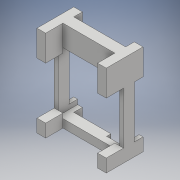
# Autodesk Inventor part: 140mmLaptopStand
Saved by Autodesk Inventor 2017 (Build 210142000, 142)
## iProperties
Created: 2016-09-13
Part Number: 140mmLaptopStand
Material: Generic
Document SubType Name: Modeling
Designer: Schmidty15
Density: 1 g/cm^3
Appearance: Default
Author: Schmidty15
Autodesk Inventor part; units mm, degrees
ref_plane "YZ Plane" through (0, 0, 0) normal (1, 0, 0) x (0, 1, 0)
ref_plane "XZ Plane" through (0, 0, 0) normal (0, 1, 0) x (-1, 0, 0)
ref_plane "XY Plane" through (0, 0, 0) normal (0, 0, 1) x (1, 0, 0)
sketch "Sketch1" plane through (0, 0, 0) normal (0, 1, 0) x (-1, 0, 0)
  line L0 (0, 0) -> (-160, 0)
  line L1 (-160, 0) -> (-160, 190)
  line L2 (-160, 190) -> (0, 190)
  line L3 (0, 190) -> (0, 0)
  dimension "d0" = 160
  dimension "d1" = 190
  constraints: 8 end point, 2 parallel, 1 horizontal, 1 perpendicular
  measures "d0" distance of L1.end L2.end
  measures "d1" distance of L0.end L1.end
extrude "Extrusion1" add sketch "Sketch1" along normal blind 55
sketch "Sketch2" plane through (0, 55, 0) normal (0, 1, 0) x (1, 0, 0)
  line L0 (0, 0) -> (10, 0)
  line L1 (10, 0) -> (10, -10)
  line L2 (10, -10) -> (0, -10)
  line L3 (0, -10) -> (0, 0)
  line L4 (10, -10) -> (150, -10)
  line L5 (150, -10) -> (150, -150)
  line L6 (150, -150) -> (10, -150)
  line L7 (10, -150) -> (10, -10)
  dimension "d4" = 10
  dimension "d5" = 10
  dimension "d6" = 140
  dimension "d7" = 140
  constraints: 16 end point, 4 parallel, 2 horizontal, 2 perpendicular
  measures "d4" distance of L1.end L2.end
  measures "d5" distance of L0.end L1.end
  measures "d6" distance of L5.end L6.end
  measures "d7" distance of L4.end L5.end
extrude "Extrusion2" cut sketch "Sketch2" against normal blind 35 contours L4 L5 L6 L7
sketch "Sketch3" plane through (0, 20, 0) normal (0, 1, 0) x (1, 0, 0)
  line L0 (10, -150) -> (10, -10) projected
  line L1 (10, -10) -> (20, -10)
  line L2 (20, -10) -> (20, -20)
  line L3 (20, -20) -> (10, -20)
  line L4 (10, -20) -> (10, -10)
  line L5 (20, -20) -> (140, -20)
  line L6 (140, -20) -> (140, -140)
  line L7 (140, -140) -> (20, -140)
  line L8 (20, -140) -> (20, -20)
  point P0 (0, 0)
  dimension "d10" = 10
  dimension "d11" = 10
  dimension "d12" = 120
  dimension "d13" = 120
  constraints: 16 end point, 4 parallel, 2 horizontal, 2 perpendicular
  measures "d10" distance of L2.end L3.end
  measures "d11" distance of L1.end L2.end
  measures "d12" distance of L6.end L7.end
  measures "d13" distance of L5.end L6.end
extrude "Extrusion3" cut sketch "Sketch3" against normal blind 20 contours L5 L6 L7 L8
sketch "Sketch4" plane through (0, 20, 0) normal (0, 1, 0) x (1, 0, 0)
  line L0 (20, -20) -> (20, -140) projected
  line L1 (20, -20) -> (10, -20)
  line L2 (10, -20) -> (10, -140)
  line L3 (10, -140) -> (20, -140)
  line L4 (20, -140) -> (20, -20)
  line L5 (140, -20) -> (20, -20) projected
  line L6 (140, -20) -> (150, -20)
  line L7 (150, -20) -> (150, -140)
  line L8 (150, -140) -> (140, -140)
  line L9 (140, -140) -> (140, -20)
  line L10 (20, -20) -> (140, -20)
  line L11 (140, -20) -> (140, -10)
  line L12 (140, -10) -> (20, -10)
  line L13 (20, -10) -> (20, -20)
  line L14 (20, -140) -> (140, -140)
  line L15 (140, -140) -> (140, -150)
  line L16 (140, -150) -> (20, -150)
  line L17 (20, -150) -> (20, -140)
  point P0 (0, 0)
  dimension "d16" = 10
  dimension "d17" = 10
  dimension "d18" = 120
  dimension "d19" = 120
  dimension "d20" = 10
  dimension "d21" = 120
  dimension "d22" = 10
  constraints: 32 end point, 8 parallel, 4 horizontal, 4 perpendicular
  measures "d16" distance of L3.end L2.end
  measures "d17" distance of L7.end L8.end
  measures "d18" distance of L6.end L7.end
  measures "d19" distance of L12.end L11.end
  measures "d20" distance of L11.end L10.end
  measures "d21" distance of L15.end L16.end
  measures "d22" distance of L14.end L15.end
extrude "Extrusion4" cut sketch "Sketch4" against normal blind 20 contours L0 L3 L2 L1 | L13 L12 L11 L5 | L14 L15 L16 L17 | L6 L7 L8 L9
sketch "Sketch5" plane through (10, 55, 150) normal (1, 0, 0) x (0, 0, -1)
  line L0 (0, -35) -> (10, -35) projected
  line L1 (10, -35) -> (130, -35)
  line L2 (130, -35) -> (130, -55)
  line L3 (130, -55) -> (10, -55)
  line L4 (10, -55) -> (10, -35)
  point P0 (150, -55)
  constraints: 8 end point, 2 parallel, 1 horizontal, 1 perpendicular
extrude "Extrusion5" cut sketch "Sketch5" against normal blind 10
sketch "Sketch6" plane through (150, 55, 10) normal (-1, 0, 0) x (0, 0, 1)
  line L0 (130, -35) -> (130, -55) projected
  line L1 (10, -35) -> (130, -35)
  line L2 (130, -35) -> (130, -55)
  line L3 (130, -55) -> (10, -55)
  line L4 (10, -55) -> (10, -35)
  point P0 (-10, -55)
  dimension "d27" = 120
  dimension "d28" = 20
  constraints: 8 end point, 2 parallel, 1 horizontal, 1 perpendicular
  measures "d27" distance of L0.end L3.end
  measures "d28" distance of L1.end L0.end
extrude "Extrusion6" cut sketch "Sketch6" against normal blind 10
sketch "Sketch7" plane through (0, 0, 0) normal (0, -1, 0) x (1, 0, 0)
  line L0 (160, 190) -> (0, 190) projected
  line L1 (160, 190) -> (150, 190)
  line L2 (150, 190) -> (150, 180)
  line L3 (150, 180) -> (160, 180)
  line L4 (160, 180) -> (160, 190)
  line L5 (0, 140) -> (20, 140) projected
  line L6 (150, 150) -> (10, 150) projected
  line L7 (0, 140) -> (20, 140)
  line L8 (20, 140) -> (20, 150)
  line L9 (20, 150) -> (0, 150)
  line L10 (0, 150) -> (0, 140)
  line L11 (10, 150) -> (10, 10) projected
  line L12 (10, 150) -> (20, 150)
  line L13 (20, 150) -> (20, 160)
  line L14 (20, 160) -> (10, 160)
  line L15 (10, 160) -> (10, 150)
  line L16 (10, 160) -> (150, 160)
  line L17 (150, 160) -> (150, 180)
  line L18 (150, 180) -> (10, 180)
  line L19 (10, 180) -> (10, 160)
  point P0 (0, 0)
  dimension "d31" = 10
  dimension "d32" = 10
  dimension "d33" = 20
  dimension "d34" = 10
  dimension "d35" = 10
  constraints: 32 end point, 8 parallel, 4 horizontal, 4 perpendicular, 1 point on line
  measures "d31" distance of L3.end L2.end
  measures "d32" distance of L2.end L1.end
  measures "d33" distance of L9.end L8.end
  measures "d34" distance of L14.end L13.end
  measures "d35" distance of L13.end L12.end
extrude "Extrusion7" cut sketch "Sketch7" against normal blind 45 contours L17 L16 L14 L19 L18
sketch "Sketch8" plane through (10, 55, 10) normal (0, 0, 1) x (1, 0, 0)
  line L0 (10, -35) -> (10, -55) projected
  line L1 (130, -55) -> (10, -55)
  line L2 (10, -55) -> (10, -35)
  line L3 (10, -35) -> (130, -35)
  line L4 (130, -35) -> (130, -55)
  point P0 (-10, -55)
  dimension "d38" = 120
  dimension "d39" = 20
  constraints: 8 end point, 2 parallel, 1 horizontal, 1 perpendicular
  measures "d38" distance of L0.start L3.end
  measures "d39" distance of L1.end L0.start
extrude "Extrusion8" cut sketch "Sketch8" against normal blind 10
sketch "Sketch9" plane through (150, 55, 10) normal (-1, 0, 0) x (0, 0, 1)
  line L0 (140, 0) -> (140, -35) projected
  line L1 (0, 0) -> (0, -35) projected
  line L2 (140, -35) -> (0, -35)
  line L3 (0, -35) -> (0, 0)
  line L4 (0, 0) -> (140, 0)
  line L5 (140, 0) -> (140, -35)
  point P0 (-10, -55)
  constraints: 8 end point, 2 parallel, 1 horizontal, 1 perpendicular
extrude "Extrusion9" cut sketch "Sketch9" against normal blind 1
sketch "Sketch10" plane through (10, 55, 150) normal (1, 0, 0) x (0, 0, -1)
  line L0 (0, 0) -> (0, -35) projected
  line L1 (0, 0) -> (140, 0)
  line L2 (140, 0) -> (140, -35)
  line L3 (140, -35) -> (0, -35)
  line L4 (0, -35) -> (0, 0)
  point P0 (150, -55)
  constraints: 8 end point, 2 parallel, 1 horizontal, 1 perpendicular
extrude "Extrusion10" cut sketch "Sketch10" against normal blind 1
sketch "Sketch11" plane through (20, 20, 10) normal (0, 0, 1) x (1, 0, 0)
  line L0 (120, 0) -> (131, 0) projected
  line L1 (131, 0) -> (-11, 0)
  line L2 (-11, 0) -> (-11, 35)
  line L3 (-11, 35) -> (131, 35)
  line L4 (131, 35) -> (131, 0)
  point P0 (-20, -20)
  constraints: 8 end point, 2 parallel, 1 horizontal, 1 perpendicular
extrude "Extrusion11" cut sketch "Sketch11" against normal blind 1
sketch "Sketch12" plane through (140, 0, 150) normal (0, 0, -1) x (-1, 0, 0)
  line L0 (-11, 55) -> (-11, 20) projected
  line L1 (-11, 55) -> (131, 55)
  line L2 (131, 55) -> (131, 20)
  line L3 (131, 20) -> (-11, 20)
  line L4 (-11, 20) -> (-11, 55)
  line L5 (0, 0) -> (-20, 0) projected
  line L6 (0, 0) -> (120, 0)
  line L7 (120, 0) -> (120, 20)
  line L8 (120, 20) -> (0, 20)
  line L9 (0, 20) -> (0, 0)
  point P0 (140, 0)
  constraints: 16 end point, 4 parallel, 2 horizontal, 2 perpendicular
extrude "Extrusion12" cut sketch "Sketch12" against normal blind 1
sketch "Sketch14" plane through (160, 55, 0) normal (0, 0, -1) x (-1, 0, 0)
  line L0 (0, -55) -> (0, 0) projected
  line L1 (20, -35) -> (20, -55) projected
  line L2 (0, -55) -> (20, -55)
  line L3 (20, -55) -> (20, -35)
  line L4 (20, -35) -> (0, -35)
  line L5 (0, -35) -> (0, -55)
  line L6 (160, -55) -> (160, -35) projected
  line L7 (140, -35) -> (140, -55) projected
  line L8 (160, -55) -> (140, -55)
  line L9 (140, -55) -> (140, -35)
  line L10 (140, -35) -> (160, -35)
  line L11 (160, -35) -> (160, -55)
  line L12 (151, -35) -> (160, -35) projected
  line L13 (160, 0) -> (0, 0) projected
  line L14 (160, -35) -> (0, -35)
  line L15 (0, -35) -> (0, 0)
  line L16 (0, 0) -> (160, 0)
  line L17 (160, 0) -> (160, -35)
  constraints: 24 end point, 6 parallel, 3 horizontal, 3 perpendicular
extrude "Extrusion13" add sketch "Sketch14" along normal blind 10
sketch "Sketch15" plane through (0, 0, 190) normal (0, 0, 1) x (1, 0, 0)
  line L0 (0, 0) -> (0, 55) projected
  line L1 (160, 0) -> (140, 0) projected
  line L2 (0, 55) -> (160, 55)
  line L3 (160, 55) -> (160, 0)
  line L4 (160, 0) -> (0, 0)
  line L5 (0, 0) -> (0, 55)
  constraints: 8 end point, 2 parallel, 1 horizontal, 1 perpendicular
extrude "Extrusion14" add sketch "Sketch15" along normal blind 10
sketch "Sketch16" plane through (0, 45, 0) normal (0, -1, 0) x (1, 0, 0)
  line L0 (10, 160) -> (10, 180) projected
  line L1 (10, 180) -> (150, 180) projected
  line L2 (10, 160) -> (150, 160)
  line L3 (150, 160) -> (150, 180)
  line L4 (150, 180) -> (10, 180)
  line L5 (10, 180) -> (10, 160)
  point P0 (0, 0)
  constraints: 8 end point, 2 parallel, 1 horizontal, 1 perpendicular
extrude "Extrusion15" add sketch "Sketch16" along normal blind 45
sketch "Sketch17" plane through (20, 20, 9) normal (0, 0, 1) x (1, 0, 0)
  line L0 (-11, 0) -> (-11, 35) projected
  line L1 (-11, 35) -> (131, 35)
  line L2 (131, 35) -> (131, 25)
  line L3 (131, 25) -> (-11, 25)
  line L4 (-11, 25) -> (-11, 35)
  point P0 (-20, -20)
  dimension "d56" = 142
  dimension "d57" = 10
  constraints: 8 end point, 2 parallel, 1 horizontal, 1 perpendicular
  measures "d56" distance of L2.end L3.end
  measures "d57" distance of L1.end L2.end
extrude "Extrusion16" cut sketch "Sketch17" against normal blind 19
sketch "Sketch19" plane through (9, 55, 150) normal (1, 0, 0) x (0, 0, -1)
  line L0 (160, 0) -> (160, -10) projected
  line L1 (141, -10) -> (160, -10) projected
  line L2 (160, 0) -> (141, 0)
  line L3 (141, 0) -> (141, -10)
  line L4 (141, -10) -> (160, -10)
  line L5 (160, -10) -> (160, 0)
  point P0 (150, -55)
  constraints: 8 end point, 2 parallel, 1 horizontal, 1 perpendicular
extrude "Extrusion17" add sketch "Sketch19" along normal blind 11
sketch "Sketch21" plane through (151, 55, 10) normal (-1, 0, 0) x (0, 0, 1)
  line L0 (-20, -10) -> (-20, 0) projected
  line L1 (-1, -10) -> (-1, -35) projected
  line L2 (-20, 0) -> (-1, 0)
  line L3 (-1, 0) -> (-1, -10)
  line L4 (-1, -10) -> (-20, -10)
  line L5 (-20, -10) -> (-20, 0)
  point P0 (-10, -55)
  constraints: 8 end point, 2 parallel, 1 horizontal, 1 perpendicular
extrude "Extrusion18" add sketch "Sketch21" along normal blind 11
sketch "Sketch22" plane through (151, 55, 10) normal (-1, 0, 0) x (0, 0, 1)
  line L0 (-1, 0) -> (141, 0) projected
  line L1 (-1, 0) -> (141, 0)
  line L2 (141, 0) -> (141, -10)
  line L3 (141, -10) -> (-1, -10)
  line L4 (-1, -10) -> (-1, 0)
  point P0 (-10, -55)
  dimension "d64" = 142
  dimension "d65" = 10
  constraints: 8 end point, 2 parallel, 1 horizontal, 1 perpendicular
  measures "d64" distance of L2.end L3.end
  measures "d65" distance of L1.end L2.end
extrude "Extrusion19" cut sketch "Sketch22" against normal blind 9
sketch "Sketch23" plane through (20, 20, 9) normal (0, 0, 1) x (1, 0, 0)
  line L0 (120, 35) -> (140, 35) projected
  line L1 (131, 25) -> (140, 25) projected
  line L2 (140, 35) -> (131, 35)
  line L3 (131, 35) -> (131, 25)
  line L4 (131, 25) -> (140, 25)
  line L5 (140, 25) -> (140, 35)
  point P0 (-20, -20)
  constraints: 8 end point, 2 parallel, 1 horizontal, 1 perpendicular
extrude "Extrusion20" add sketch "Sketch23" along normal blind 11
sketch "Sketch24" plane through (9, 55, 150) normal (1, 0, 0) x (0, 0, -1)
  line L0 (-1, 0) -> (141, 0) projected
  line L1 (141, 0) -> (-1, 0)
  line L2 (-1, 0) -> (-1, -10)
  line L3 (-1, -10) -> (141, -10)
  line L4 (141, -10) -> (141, 0)
  point P0 (150, -55)
  dimension "d70" = 142
  dimension "d71" = 10
  constraints: 8 end point, 2 parallel, 1 horizontal, 1 perpendicular
  measures "d70" distance of L3.end L2.end
  measures "d71" distance of L2.end L1.end
extrude "Extrusion21" cut sketch "Sketch24" against normal blind 9
sketch "Sketch25" plane through (20, 20, 9) normal (0, 0, 1) x (1, 0, 0)
  line L0 (-20, 25) -> (-20, 35) projected
  line L1 (-11, 0) -> (-11, 25) projected
  line L2 (-20, 35) -> (-11, 35)
  line L3 (-11, 35) -> (-11, 25)
  line L4 (-11, 25) -> (-20, 25)
  line L5 (-20, 25) -> (-20, 35)
  point P0 (-20, -20)
  constraints: 8 end point, 2 parallel, 1 horizontal, 1 perpendicular
extrude "Extrusion22" add sketch "Sketch25" along normal blind 11
sketch "Sketch26" plane through (140, 0, 151) normal (0, 0, -1) x (-1, 0, 0)
  line L0 (-20, 45) -> (-20, 55) projected
  line L1 (-11, 45) -> (-20, 45) projected
  line L2 (-20, 55) -> (-11, 55)
  line L3 (-11, 55) -> (-11, 45)
  line L4 (-11, 45) -> (-20, 45)
  line L5 (-20, 45) -> (-20, 55)
  line L6 (-20, 55) -> (140, 55) projected
  line L7 (131, 45) -> (140, 45) projected
  line L8 (140, 55) -> (131, 55)
  line L9 (131, 55) -> (131, 45)
  line L10 (131, 45) -> (140, 45)
  line L11 (140, 45) -> (140, 55)
  point P0 (140, 0)
  constraints: 16 end point, 4 parallel, 2 horizontal, 2 perpendicular
extrude "Extrusion23" add sketch "Sketch26" along normal blind 11
sketch "Sketch27" plane through (140, 0, 151) normal (0, 0, -1) x (-1, 0, 0)
  line L0 (0, 0) -> (0, 20) projected
  line L1 (120, 0) -> (0, 0) projected
  line L2 (0, 20) -> (120, 20)
  line L3 (120, 20) -> (120, 0)
  line L4 (120, 0) -> (0, 0)
  line L5 (0, 0) -> (0, 20)
  point P0 (140, 0)
  constraints: 8 end point, 2 parallel, 1 horizontal, 1 perpendicular
extrude "Extrusion24" cut sketch "Sketch27" against normal blind 50
sketch "Sketch28" plane through (140, 0, 151) normal (0, 0, -1) x (-1, 0, 0)
  line L0 (-11, 20) -> (-11, 55) projected
  line L1 (-11, 55) -> (0, 55)
  line L2 (-11, 55) -> (131, 55) projected
  line L3 (131, 55) -> (120, 55)
  line L4 (0, 55) -> (120, 55)
  line L5 (120, 55) -> (120, 45)
  line L6 (120, 45) -> (0, 45)
  line L7 (0, 45) -> (0, 55)
  point P0 (140, 0)
  dimension "d80" = 11
  dimension "d81" = 11
  dimension "d82" = 120
  dimension "d83" = 10
  constraints: 12 end point, 2 parallel, 2 point on line, 1 horizontal, 1 perpendicular
  measures "d80" distance of L0.end L1.end
  measures "d81" distance of L2.end L3.end
  measures "d82" distance of L5.end L6.end
  measures "d83" distance of L4.end L5.end
extrude "Extrusion25" cut sketch "Sketch28" against normal blind 50
sketch "Sketch29" plane through (20, 20, 9) normal (0, 0, 1) x (1, 0, 0)
  line L0 (120, 25) -> (86, 25)
  line L1 (120, 25) -> (0, 25) projected
  line L2 (86, 25) -> (106, 25)
  line L3 (106, 25) -> (106, 15)
  line L4 (106, 15) -> (86, 15)
  line L5 (86, 15) -> (86, 25)
  point P0 (-20, -20)
  dimension "d86" = 34
  dimension "d87" = 20
  dimension "d88" = 10
  constraints: 10 end point, 2 parallel, 1 horizontal, 1 perpendicular, 1 point on line
  measures "d86" distance of L0.start L0.end
  measures "d87" distance of L3.end L4.end
  measures "d88" distance of L2.end L3.end
extrude "Extrusion26" cut sketch "Sketch29" against normal blind 19
sketch "Sketch30" plane through (20, 20, 9) normal (0, 0, 1) x (1, 0, 0)
  line L0 (120, 25) -> (106, 25) projected
  line L1 (106, 15) -> (86, 15) projected
  line L2 (120, 25) -> (106, 25)
  line L3 (106, 25) -> (106, 15)
  line L4 (106, 15) -> (120, 15)
  line L5 (120, 15) -> (120, 25)
  point P0 (-20, -20)
  constraints: 8 end point, 2 parallel, 1 horizontal, 1 perpendicular
extrude "Extrusion27" cut sketch "Sketch30" against normal blind 19
sketch "Sketch31" plane through (0, 0, 0) normal (0, -1, 0) x (1, 0, 0)
  line L0 (0, 20) -> (0, -10) projected
  line L1 (20, 20) -> (20, 9) projected
  line L2 (0, -10) -> (20, -10)
  line L3 (20, -10) -> (20, 20)
  line L4 (20, 20) -> (0, 20)
  line L5 (0, 20) -> (0, -10)
  line L6 (106, -10) -> (140, -10) projected
  line L7 (160, -10) -> (160, 20) projected
  line L8 (140, -10) -> (160, -10)
  line L9 (160, -10) -> (160, 20)
  line L10 (160, 20) -> (140, 20)
  line L11 (140, 20) -> (140, -10)
  line L12 (151, 140) -> (140, 140) projected
  line L13 (160, 140) -> (160, 200) projected
  line L14 (140, 140) -> (160, 140)
  line L15 (160, 140) -> (160, 200)
  line L16 (160, 200) -> (140, 200)
  line L17 (140, 200) -> (140, 140)
  line L18 (0, 200) -> (0, 140) projected
  line L19 (20, 200) -> (0, 200) projected
  line L20 (0, 140) -> (20, 140)
  line L21 (20, 140) -> (20, 200)
  line L22 (20, 200) -> (0, 200)
  line L23 (0, 200) -> (0, 140)
  point P0 (0, 0)
  constraints: 32 end point, 8 parallel, 4 horizontal, 4 perpendicular
extrude "Extrusion28" add sketch "Sketch31" along normal blind 20
sketch "Sketch32" plane through (0, 55, 0) normal (0, 1, 0) x (1, 0, 0)
  line L0 (0, -20) -> (0, 10) projected
  line L1 (20, -9) -> (20, 10) projected
  line L2 (0, 10) -> (20, 10)
  line L3 (20, 10) -> (20, -9)
  line L4 (20, -9) -> (0, -9)
  line L5 (0, -9) -> (0, 10)
  line L6 (9, -9) -> (9, -20) projected
  line L7 (9, -20) -> (0, -20)
  line L8 (0, -20) -> (0, -9)
  line L9 (0, -9) -> (9, -9)
  line L10 (9, -9) -> (9, -20)
  line L11 (151, -20) -> (151, -9) projected
  line L12 (160, 10) -> (160, -20) projected
  line L13 (151, -20) -> (160, -20)
  line L14 (160, -20) -> (160, 10)
  line L15 (160, 10) -> (151, 10)
  line L16 (151, 10) -> (151, -20)
  line L17 (151, 10) -> (140, 10)
  line L18 (140, 10) -> (140, -9)
  line L19 (140, -9) -> (151, -9)
  line L20 (151, -9) -> (151, 10)
  line L21 (160, -200) -> (140, -200) projected
  line L22 (140, -140) -> (140, -151) projected
  line L23 (160, -200) -> (140, -200)
  line L24 (140, -200) -> (140, -151)
  line L25 (140, -151) -> (160, -151)
  line L26 (160, -151) -> (160, -200)
  line L27 (151, -151) -> (151, -140) projected
  line L28 (160, -140) -> (160, -200) projected
  line L29 (151, -151) -> (160, -151)
  line L30 (160, -151) -> (160, -140)
  line L31 (160, -140) -> (151, -140)
  line L32 (151, -140) -> (151, -151)
  line L33 (0, -140) -> (20, -140) projected
  line L34 (9, -151) -> (20, -151) projected
  line L35 (0, -140) -> (9, -140)
  line L36 (9, -140) -> (9, -151)
  line L37 (9, -151) -> (0, -151)
  line L38 (0, -151) -> (0, -140)
  line L39 (20, -151) -> (20, -200) projected
  line L40 (20, -200) -> (0, -200)
  line L41 (0, -200) -> (0, -151)
  line L42 (0, -151) -> (20, -151)
  line L43 (20, -151) -> (20, -200)
  point P0 (0, 0)
  constraints: 64 end point, 16 parallel, 8 horizontal, 8 perpendicular, 1 point on line
extrude "Extrusion29" add sketch "Sketch32" along normal blind 10
body "Solid1"
